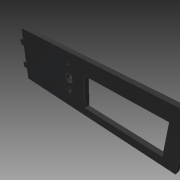
# Autodesk Inventor part: front_panel_2004_display
Saved by Autodesk Inventor 2014 (Build 180170000, 170)
## iProperties
Created: 2014-01-11
Part Number: front_panel_2004_display
Material: Generic
Document SubType Name: Modeling
Designer: buben
Density: 1 g/cm^3
Appearance: Anodized - Dark Gray
Author: buben
Autodesk Inventor part; units mm, degrees
ref_plane "YZ Plane" through (0, 0, 0) normal (1, 0, 0) x (0, 1, 0)
ref_plane "XZ Plane" through (0, 0, 0) normal (0, 1, 0) x (-1, 0, 0)
ref_plane "XY Plane" through (0, 0, 0) normal (0, 0, 1) x (1, 0, 0)
sketch "Sketch1" plane through (0, 0, 0) normal (0, 1, 0) x (-1, 0, 0)
  line L0 (0, 0) -> (220, 0)
  line L1 (220, 0) -> (220, 70)
  line L2 (220, 70) -> (0, 70)
  line L3 (0, 70) -> (0, 0)
  line L4 (16, 51) -> (114, 51) construction
  line L5 (114, 51) -> (114, 11) construction
  line L6 (114, 11) -> (16, 11) construction
  line L7 (16, 11) -> (16, 51) construction
  line L8 (15.5, 51.5) -> (114.5, 51.5)
  line L9 (114.5, 51.5) -> (114.5, 10.5)
  line L10 (114.5, 10.5) -> (15.5, 10.5)
  line L11 (15.5, 10.5) -> (15.5, 51.5)
  circle A0 centre (139, 55) radius 1.5
  circle A1 centre (139, 37.5) radius 5.5
  circle A2 centre (139, 22) radius 3
  line L12 (2, 65) -> (152, 65) construction
  line L13 (152, 65) -> (152, 10) construction
  line L14 (152, 10) -> (2, 10) construction
  line L15 (2, 10) -> (2, 65) construction
  point P0 (65, 51.5)
  point P1 (65, 51)
  point P2 (114, 31)
  point P3 (114.5, 31)
  dimension "d11" = 220
  dimension "d106" = 40
  dimension "d107" = 98
  dimension "d108" = 99
  dimension "d109" = 41
  dimension "d110" = 25
  dimension "d111" = 6
  dimension "d112" = 15.5
  dimension "d113" = 17.5
  dimension "d114" = 13.5
  dimension "d115" = 3
  dimension "d116" = 11
  dimension "d117" = 55
  dimension "d118" = 150
  dimension "d119" = 14
  dimension "d120" = 14
  dimension "d121" = 5
  dimension "d122" = 2
  dimension "d123" = 10
  constraints: 32 end point, 8 parallel, 4 horizontal, 4 midpoint, 4 perpendicular, 3 centre point, 3 vertical alignment, 1 horizontal alignment
  measures "d11" distance of L0.start L0.end
  measures "d106" distance of L5.start L5.end
  measures "d107" distance of L5.end L7.start
  measures "d108" distance of L9.end L10.end
  measures "d109" distance of L9.start L9.end
  measures "d110" distance from line of A1.centre L5
  measures "d111" diameter of A2
  measures "d112" distance of A2.centre A1.centre
  measures "d113" distance of A0.centre A1.centre
  measures "d114" distance from line of A1.centre L4
  measures "d115" diameter of A0
  measures "d116" diameter of A1
  measures "d117" distance of L15.start L15.end
  measures "d118" distance of L15.end L13.start
  measures "d119" distance between parallel lines of L7 L15
  measures "d120" distance between parallel lines of L12 L4
  measures "d121" distance between parallel lines of L2 L12
  measures "d122" distance between parallel lines of L3 L15
  measures "d123" distance between parallel lines of L0 L14
extrude "Extrusion8" add sketch "Sketch1" along normal blind 6
sketch "Sketch7" plane through (0, 6, 0) normal (0, 1, 0) x (1, 0, 0)
  line L0 (0, 0) -> (-220, 0) projected
  line L1 (-220, 0) -> (-220, -70) projected
  line L2 (-220, -70) -> (0, -70) projected
  line L3 (0, -70) -> (0, 0) projected
  line L4 (-220, -15) -> (-224, -15)
  line L5 (-226, -17) -> (-226, -21)
  line L6 (-224, -23) -> (-220, -23)
  line L7 (-220, -23) -> (-220, -15)
  line L8 (-220, -47) -> (-224, -47)
  line L9 (-226, -49) -> (-226, -53)
  line L10 (-224, -55) -> (-220, -55)
  line L11 (-220, -55) -> (-220, -47)
  line L12 (0, -15) -> (4, -15)
  line L13 (6, -17) -> (6, -21)
  line L14 (4, -23) -> (0, -23)
  line L15 (0, -23) -> (0, -15)
  line L16 (0, -47) -> (4, -47)
  line L17 (6, -49) -> (6, -53)
  line L18 (4, -55) -> (0, -55)
  line L19 (0, -55) -> (0, -47)
  arc A0 (-224, -15) -> (-226, -17) centre (-224, -17) ccw
  arc A1 (-226, -21) -> (-224, -23) centre (-224, -21) ccw
  arc A2 (-224, -47) -> (-226, -49) centre (-224, -49) ccw
  arc A3 (-226, -53) -> (-224, -55) centre (-224, -53) ccw
  arc A4 (6, -17) -> (4, -15) centre (4, -17) ccw
  arc A5 (4, -23) -> (6, -21) centre (4, -21) ccw
  arc A6 (6, -49) -> (4, -47) centre (4, -49) ccw
  arc A7 (4, -55) -> (6, -53) centre (4, -53) ccw
  dimension "d126" = 2
  dimension "d127" = 15
  dimension "d128" = 8
  dimension "d129" = 8
  dimension "d130" = 15
  dimension "d131" = 6
  dimension "d132" = 6
  constraints: 32 end point, 16 point on circle, 16 tangent, 8 centre point, 8 parallel, 7 equal radius, 6 collinear, 4 horizontal, 4 perpendicular, 4 point on line
  measures "d126" radius of A0
  measures "d127" distance between parallel lines of L0 L4
  measures "d128" distance between parallel lines of L6 L4
  measures "d129" distance between parallel lines of L10 L8
  measures "d130" distance between parallel lines of L2 L10
  measures "d131" distance between parallel lines of L1 L5
  measures "d132" distance between parallel lines of L3 L13
extrude "Extrusion9" add sketch "Sketch7" against normal blind 6 contours L12 A4 L13 A5 L14 L3 | L1 L6 A1 L5 A0 L4 | L16 A6 L17 A7 L18 L3 | L1 L10 A3 L9 A2 L8
body "Solid3"
